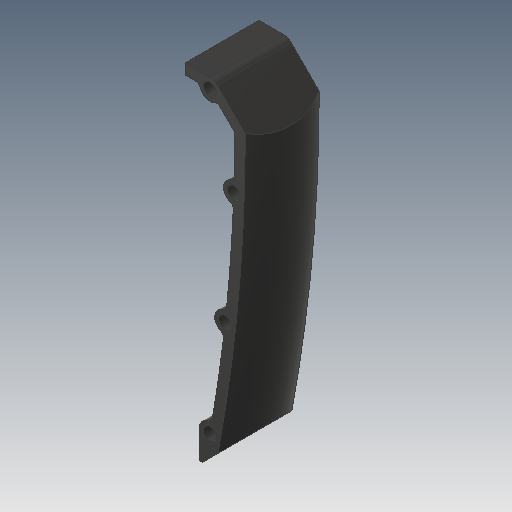
# Autodesk Inventor part: Handler
Saved by Autodesk Inventor 2019.4 (Build 234330000, 330)
## iProperties
Created: 2019-01-12
Part Number: Handler
Material: 一般
Document SubType Name: Modeling
Designer: y6tada
Density: 1 g/cm^3
Appearance: 滑らか - 黒
Mass: 24.3287 g
Surface Area: 114.561 cm^2
Volume: 24.3287 cm^3
Author: y6tada
Autodesk Inventor part; units mm, degrees
ref_plane "YZ Plane" through (0, 0, 0) normal (1, 0, 0) x (0, 1, 0)
ref_plane "XZ Plane" through (0, 0, 0) normal (0, 1, 0) x (-1, 0, 0)
sketch "スケッチ1" plane through (0, 0, 0) normal (0, 0, 1) x (1, 0, 0)
  line L0 (40.5687, 65) -> (31, 65) projected
  arc A0 (43.3971, 63.8284) -> (40.5687, 65) centre (40.5687, 61) ccw projected
  line L1 (54.2256, 53) -> (43.3971, 63.8284) projected
  arc A1 (43.6795, -59) -> (54.2256, 53) centre (-545.7744, 53) ccw construction
  line L2 (37.6795, -65) -> (43.6795, -59) projected
  circle A2 centre (40.542, -54) radius 1.3 construction
  circle A3 centre (46.4476, -14) radius 1.3 construction
  circle A4 centre (49.8194, 31) radius 1.3 construction
  circle A5 centre (40.5687, 61) radius 1.3 construction
  line L3 (36.542, -54) -> (36.542, -65)
  line L4 (36.542, -65) -> (37.6795, -65)
  arc A6 (36.607, -53.2819) -> (46.2163, 49.6955) centre (-545.7744, 53) ccw construction
  line L5 (46.2163, 49.6955) -> (38.9118, 57) construction
  line L6 (38.9118, 57) -> (31, 57) construction
  line L7 (31, 65) -> (31, 61)
  arc A7 (40.1421, -50.02) -> (36.542, -54) centre (40.542, -54) ccw
  circle A8 centre (40.5687, 61) radius 1.5
  circle A9 centre (49.8194, 31) radius 1.5
  circle A10 centre (46.4476, -14) radius 1.5
  circle A11 centre (40.542, -54) radius 1.5
  arc A12 (49.9078, -52.7717) -> (59.2051, 48.0205) centre (-545.7744, 53) ccw
  line L8 (54.2256, 53) -> (59.2051, 48.0205)
  line L9 (43.6795, -59) -> (49.9078, -52.7717)
  arc A13 (45.7787, -10.0563) -> (44.9146, -17.6946) centre (46.4476, -14) ccw
  arc A14 (41.47, -48.7837) -> (45.8287, -19.2619) centre (-545.7744, 53) ccw
  arc A15 (48.854, 34.8818) -> (48.5703, 27.2) centre (49.8194, 31) ccw
  arc A16 (47.0198, -8.7328) -> (49.6003, 25.7064) centre (-545.7744, 53) ccw
  arc A17 (49.9914, 36.2954) -> (50.2212, 50.7204) centre (-545.7744, 53) ccw
  arc A18 (36.7203, 59.9091) -> (42.5185, 57.5074) centre (40.5687, 61) ccw
  line L10 (35.2772, 61) -> (31, 61)
  line L11 (49.7819, 51.7868) -> (44.3104, 57.2583)
  line L12 (31, 61) -> (31, 57) construction
  arc A19 (36.7203, 59.9091) -> (35.2772, 61) centre (35.2772, 59.5) ccw
  arc A20 (44.3104, 57.2583) -> (42.5185, 57.5074) centre (43.2497, 56.1977) ccw
  arc A21 (50.2212, 50.7204) -> (49.7819, 51.7868) centre (48.7212, 50.7262) ccw
  arc A22 (48.854, 34.8818) -> (49.9914, 36.2954) centre (48.492, 36.3374) ccw
  arc A23 (49.6003, 25.7064) -> (48.5703, 27.2) centre (48.1019, 25.7751) ccw
  arc A24 (45.7787, -10.0563) -> (47.0198, -8.7328) centre (45.5279, -8.5774) ccw
  arc A25 (45.8287, -19.2619) -> (44.9146, -17.6946) centre (44.3397, -19.08) ccw
  arc A26 (40.1421, -50.02) -> (41.47, -48.7837) centre (39.9921, -48.5276) ccw
  point P0 (0, 0)
  point P1 (50.2233, 51.3454)
  point P2 (36.5687, 61)
  point P3 (43.3971, 58.1716)
  dimension "d1" = 8
  dimension "d2" = 4
  dimension "d3" = 3
  dimension "d6" = 5
  dimension "d48" = 4
  dimension "d50" = 4
  dimension "d51" = 4
  dimension "d52" = 1.5
  dimension "d53" = 4
  constraints: 38 point on circle, 21 centre point, 20 end point, 18 tangent, 15 equal radius, 6 coincident, 3 point on line, 3 vertical, 2 collinear, 2 parallel, 1 concentric, 1 perpendicular, 2 other
  measures "d1" distance of L0.end L6.end
  measures "d2" radius of A7
  measures "d3" diameter of A8
  measures "d6" radial gap between concentric circles of A12 A1
  measures "d48" radial gap between concentric circles of A14 A6
  measures "d50" distance between parallel lines of L5 L11
  measures "d51" distance of L0.end L7.end
  measures "d52" radius of A19
  measures "d53" distance from line of L3 A2.centre
extrude "押し出し1" add sketch "スケッチ1" along normal blind 14.25
ref_plane "作業平面1" through (31, 53, 0) normal (0, 1, 0) x (1, 0, 0)
sketch "スケッチ4" plane through (31, 53, 0) normal (0, 1, 0) x (1, 0, 0)
  line L0 (23.2256, -14.25) -> (23.2256, -17.25) construction
  line L1 (23.2256, -14.25) -> (23.2256, 0) construction
  line L2 (23.2256, 0) -> (26.2256, 0) construction
  arc A0 (23.2256, -14.25) -> (26.2256, 0) centre (-9.1182, 0) ccw
  line L3 (26.2256, 0) -> (31.2256, 0)
  line L4 (31.2256, 0) -> (31.2256, -14.25)
  line L5 (31.2256, -14.25) -> (23.2256, -14.25)
  line L6 (-576.7744, 3.45) -> (-576.7744, -20.7) projected
  point P0 (-31, 0)
  dimension "d30" = 3
  dimension "d31" = 8
  constraints: 10 end point, 2 horizontal, 2 perpendicular, 2 point on circle, 2 point on line, 1 centre point, 1 vertical
  measures "d30" distance of L1.end L2.end
  measures "d31" distance of L4.end L0.start
revolve "回転1" cut sketch "スケッチ4" angle 20 about axis through (-545.7744, 53, 0) along (0, 0, -1)
sketch "スケッチ2" plane through (0, 0, 0) normal (0, 0, 1) x (1, 0, 0)
  line L0 (54.0259, 37.5243) -> (75.618, 31.7388)
  line L1 (46.8746, -40.6329) -> (69.444, -38.252)
  arc A0 (46.8746, -40.6329) -> (54.0259, 37.5243) centre (-545.7744, 53) ccw
  arc A1 (56.0777, -25.8862) -> (60.4183, 21.7048) centre (-545.7744, 53) ccw
  line L2 (69.6232, 22.9923) -> (64.1907, 24.4479)
  line L3 (65.0021, -28.6651) -> (59.367, -29.2596)
  arc A2 (64.1907, 24.4479) -> (60.4183, 21.7048) centre (63.4143, 21.5502) ccw
  arc A3 (56.0777, -25.8862) -> (59.367, -29.2596) centre (59.0522, -26.2761) ccw
  line L4 (-545.7744, 53) -> (54.0259, 37.5243) construction
  line L5 (46.8746, -40.6329) -> (-545.7744, 53) construction
  arc A4 (43.6795, -59) -> (54.2256, 53) centre (-545.7744, 53) ccw construction
  arc A5 (76.5322, -31.3709) -> (81.5387, 23.6373) centre (-545.7744, 53) ccw
  arc A6 (69.444, -38.252) -> (76.5322, -31.3709) centre (68.6047, -30.2962) ccw
  arc A7 (81.5387, 23.6373) -> (75.618, 31.7388) centre (73.5475, 24.0114) ccw
  arc A8 (68.4245, -25.8002) -> (72.5681, 19.5265) centre (-46.8367, 7.5894) ccw
  line L6 (-545.7744, 53) -> (79.6405, -3.9219) construction
  arc A9 (68.8779, -35.5633) -> (74.7819, 29.53) centre (-545.7744, 53) ccw construction
  arc A10 (72.5681, 19.5265) -> (69.6232, 22.9923) centre (68.5879, 19.1286) ccw
  arc A11 (65.0021, -28.6651) -> (68.4245, -25.8002) centre (64.5824, -24.6872) ccw
  line L7 (40.5687, 65) -> (31, 65) projected
  point P0 (0, 0)
  point P1 (81.8072, 30.0804)
  point P2 (75.6564, -37.5967)
  point P3 (72.26, 22.2858)
  point P4 (67.6436, -28.3864)
  dimension "d7" = 7
  dimension "d9" = 3
  dimension "d11" = 15
  dimension "d12" = 10
  dimension "d13" = 10
  dimension "d14" = 7.5
  dimension "d38" = 21
  dimension "d41" = 8
  dimension "d42" = 7
  dimension "d43" = 4
  dimension "d44" = 120
  dimension "d45" = 15
  dimension "d46" = 15
  constraints: 28 point on circle, 14 end point, 13 tangent, 11 centre point, 7 point on line, 4 equal radius, 2 parallel, 1 concentric
  measures "d7" radial gap between concentric circles of A0 A1
  measures "d9" radius of A2
  measures "d11" distance from line of A4.end L0
  measures "d12" distance between parallel lines of L1 L3
  measures "d13" distance between parallel lines of L0 L2
  measures "d14" angle of L4 L5
  measures "d38" radial gap between concentric circles of A1 A5
  measures "d41" radius of A6
  measures "d42" radial gap between concentric circles of A5 A9
  measures "d43" radius of A10
  measures "d44" radius of A8
  measures "d45" angle of L1 L5
  measures "d46" angle of L7 L0
extrude "押し出し2" [suppressed]
fillet "フィレット1" [suppressed]
sketch "スケッチ5" plane through (0, 0, 14.25) normal (0, 0, 1) x (1, 0, 0)
  circle A0 centre (40.5687, 61) radius 1.5 construction
  circle A1 centre (40.5687, 61) radius 2.5
  circle A2 centre (49.8194, 31) radius 1.5 construction
  circle A3 centre (46.4476, -14) radius 1.5 construction
  circle A4 centre (40.542, -54) radius 1.5 construction
  circle A5 centre (49.8194, 31) radius 2.5
  circle A6 centre (46.4476, -14) radius 2.5
  circle A7 centre (40.542, -54) radius 2.5
  point P0 (0, 0)
  dimension "d35" = 5
  constraints: 4 centre point, 4 coincident, 3 equal radius
  measures "d35" diameter of A1
extrude "押し出し3" cut sketch "スケッチ5" against normal blind 5
mirror "ミラー1" about plane through (0, 0, 0) normal (0, 0, 1) of "押し出し1", "回転1", "押し出し3"
